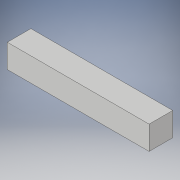
# Autodesk Inventor part: 2x2 Beam Test
Saved by Autodesk Inventor 2018 (Build 220112000, 112)
## iProperties
Created: 2018-12-05
Part Number: 2x2 Beam Test
Material: Generic
Document SubType Name: Modeling
Designer: gbgic
Density: 1 g/cm^3
Appearance: Default
Author: gbgic
Autodesk Inventor part; units mm, degrees
ref_plane "YZ Plane" through (0, 0, 0) normal (1, 0, 0) x (0, 1, 0)
ref_plane "XZ Plane" through (0, 0, 0) normal (0, 1, 0) x (-1, 0, 0)
ref_plane "XY Plane" through (0, 0, 0) normal (0, 0, 1) x (1, 0, 0)
sketch "Sketch1" plane through (0, 0, 0) normal (1, 0, 0) x (0, 1, 0)
  line L0 (29.7311, 5.6909) -> (-21.0689, 5.6909)
  line L1 (-21.0689, 5.6909) -> (-21.0689, -45.1091)
  line L2 (-21.0689, -45.1091) -> (29.7311, -45.1091)
  line L3 (29.7311, -45.1091) -> (29.7311, 5.6909)
  point P0 (0, 0)
  dimension "d0" = 50.8
  dimension "d1" = 50.8
  constraints: 8 end point, 2 parallel, 1 horizontal, 1 perpendicular
  measures "d0" distance of L2.end L1.end
  measures "d1" distance of L1.end L0.end
extrude "Extrusion1" add sketch "Sketch1" along normal blind 304.8
body "Solid1"
